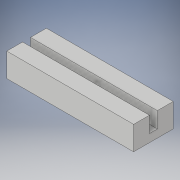
# Autodesk Inventor part: Test1
Saved by Autodesk Inventor 2018.2 (Build 222227000, 227)
## iProperties
Created: 2018-03-28
Part Number: Test1
Material: Generic
Document SubType Name: Modeling
Designer: martin
Density: 1 g/cm^3
Appearance: Default
Author: martin
Autodesk Inventor part; units mm, degrees
ref_plane "YZ Plane" through (0, 0, 0) normal (1, 0, 0) x (0, 1, 0)
ref_plane "XZ Plane" through (0, 0, 0) normal (0, 1, 0) x (-1, 0, 0)
ref_plane "XY Plane" through (0, 0, 0) normal (0, 0, 1) x (1, 0, 0)
sketch "Sketch1" plane through (0, 0, 0) normal (0, 1, 0) x (-1, 0, 0)
  line L0 (-25.4, -7.9375) -> (25.4, -7.9375)
  line L1 (25.4, -7.9375) -> (25.4, 7.9375)
  line L2 (25.4, 7.9375) -> (-25.4, 7.9375)
  line L3 (-25.4, 7.9375) -> (-25.4, -7.9375)
  line L4 (-25.4, -7.9375) -> (25.4, 7.9375) construction
  line L5 (25.4, -7.9375) -> (-25.4, 7.9375) construction
  point P0 (0, 0)
  dimension "d0" = 50.8
  dimension "d1" = 15.875
  constraints: 12 end point, 2 midpoint, 2 parallel, 1 horizontal, 1 perpendicular
  measures "d0" distance of L0.start L0.end
  measures "d1" distance of L0.end L1.end
extrude "Extrusion1" add sketch "Sketch1" along normal blind 9.525
sketch "Sketch2" plane through (-25.4, 0, -7.9375) normal (-1, 0, 0) x (0, 0, 1)
  line L0 (0, 9.525) -> (15.875, 9.525) projected
  line L1 (9.5418, 3.175) -> (6.3668, 3.175)
  line L2 (6.3668, 3.175) -> (6.3668, 9.525)
  line L3 (6.3668, 9.525) -> (9.5418, 9.525)
  line L4 (9.5418, 9.525) -> (9.5418, 3.175)
  line L5 (9.5418, 3.175) -> (6.3668, 9.525) construction
  line L6 (6.3668, 3.175) -> (9.5418, 9.525) construction
  point P0 (7.9375, 0)
  point P1 (7.9543, 6.35)
  dimension "d4" = 3.175
  dimension "d5" = 6.35
  constraints: 12 end point, 2 midpoint, 2 parallel, 1 horizontal, 1 perpendicular, 1 point on line
  measures "d4" distance of L1.start L1.end
  measures "d5" distance of L3.end L1.start
extrude "Extrusion2" cut sketch "Sketch2" against normal up to next
body "Solid1"
